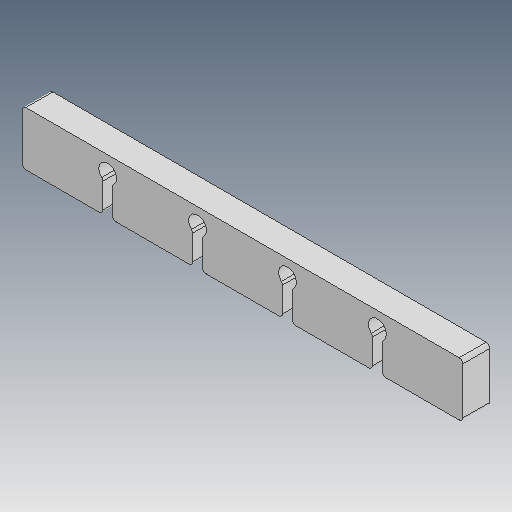
# Autodesk Inventor part: SlipersLåda 211018007
Saved by Autodesk Inventor 2020 (Build 240168000, 168)
## iProperties
Created: 2021-10-19
Part Number: SlipersLåda 211018007
Material: Generic
Document SubType Name: Modeling
Designer: dicpet001
Density: 1 g/cm^3
Appearance: Default
Author: dicpet001
Autodesk Inventor part; units mm, degrees
ref_plane "YZ Plane" through (0, 0, 0) normal (1, 0, 0) x (0, 1, 0)
ref_plane "XZ Plane" through (0, 0, 0) normal (0, 1, 0) x (-1, 0, 0)
ref_plane "XY Plane" through (0, 0, 0) normal (0, 0, 1) x (1, 0, 0)
sketch "Sketch1" plane through (0, 0, 0) normal (0, 0, 1) x (1, 0, 0)
  line L0 (0, 21.5799) -> (0, -21.5799) projected
  line L1 (-172.0799, 0) -> (172.0799, 0) projected
  line L2 (-120.5, 15) -> (120.5, 15)
  line L3 (122.5, 13) -> (122.5, -13)
  line L4 (-122.5, -13) -> (-122.5, 13)
  arc A0 (-21.6071, 2.3273) -> (-28.3929, 2.3273) centre (-25, 6) ccw
  line L5 (-25, 6) -> (-25, -2.9295)
  line L6 (-27.75, 0.8583) -> (-27.75, -13)
  line L7 (-22.25, 0.8583) -> (-22.25, -13)
  arc A1 (-27.75, 0.8583) -> (-28.3929, 2.3273) centre (-29.75, 0.8583) ccw
  arc A2 (-21.6071, 2.3273) -> (-22.25, 0.8583) centre (-20.25, 0.8583) ccw
  arc A3 (-29.75, -15) -> (-27.75, -13) centre (-29.75, -13) ccw
  arc A4 (-22.25, -13) -> (-20.25, -15) centre (-20.25, -13) ccw
  arc A5 (-71.6071, 2.3273) -> (-78.3929, 2.3273) centre (-75, 6) ccw
  line L8 (-75, 6) -> (-75, -2.9295)
  line L9 (-77.75, 0.8583) -> (-77.75, -13)
  line L10 (-72.25, 0.8583) -> (-72.25, -13)
  arc A6 (-77.75, 0.8583) -> (-78.3929, 2.3273) centre (-79.75, 0.8583) ccw
  arc A7 (-71.6071, 2.3273) -> (-72.25, 0.8583) centre (-70.25, 0.8583) ccw
  arc A8 (-79.75, -15) -> (-77.75, -13) centre (-79.75, -13) ccw
  arc A9 (-72.25, -13) -> (-70.25, -15) centre (-70.25, -13) ccw
  line L11 (-29.75, -15) -> (-70.25, -15)
  line L12 (-79.75, -15) -> (-120.5, -15)
  arc A10 (28.3929, 2.3273) -> (21.6071, 2.3273) centre (25, 6) ccw
  line L13 (25, 6) -> (25, -2.9295)
  line L14 (27.75, 0.8583) -> (27.75, -13)
  line L15 (22.25, 0.8583) -> (22.25, -13)
  arc A11 (28.3929, 2.3273) -> (27.75, 0.8583) centre (29.75, 0.8583) ccw
  arc A12 (22.25, 0.8583) -> (21.6071, 2.3273) centre (20.25, 0.8583) ccw
  arc A13 (27.75, -13) -> (29.75, -15) centre (29.75, -13) ccw
  arc A14 (20.25, -15) -> (22.25, -13) centre (20.25, -13) ccw
  line L16 (72.25, 0.8583) -> (72.25, -13)
  arc A15 (72.25, 0.8583) -> (71.6071, 2.3273) centre (70.25, 0.8583) ccw
  arc A16 (70.25, -15) -> (72.25, -13) centre (70.25, -13) ccw
  arc A17 (78.3929, 2.3273) -> (71.6071, 2.3273) centre (75, 6) ccw
  line L17 (77.75, 0.8583) -> (77.75, -13)
  arc A18 (78.3929, 2.3273) -> (77.75, 0.8583) centre (79.75, 0.8583) ccw
  line L18 (75, 6) -> (75, -2.9295)
  arc A19 (77.75, -13) -> (79.75, -15) centre (79.75, -13) ccw
  line L19 (20.25, -15) -> (-20.25, -15)
  line L20 (120.5, -15) -> (79.75, -15)
  line L21 (70.25, -15) -> (29.75, -15)
  arc A20 (-120.5, 15) -> (-122.5, 13) centre (-120.5, 13) ccw
  arc A21 (-122.5, -13) -> (-120.5, -15) centre (-120.5, -13) ccw
  arc A22 (120.5, -15) -> (122.5, -13) centre (120.5, -13) ccw
  arc A23 (122.5, 13) -> (120.5, 15) centre (120.5, 13) ccw
  point P0 (0, 0)
  point P1 (-122.5, 15)
  point P2 (122.5, 15)
  point P3 (-122.5, -15)
  point P4 (-27.75, 1.8242)
  point P5 (-22.25, 1.8242)
  point P6 (-77.75, 1.8242)
  point P7 (-72.25, 1.8242)
  point P8 (27.75, 1.8242)
  point P9 (22.25, 1.8242)
  point P10 (72.25, 1.8242)
  point P11 (77.75, 1.8242)
  dimension "d0" = 245
  dimension "d1" = 30
  dimension "d2" = 10
  dimension "d3" = 25
  dimension "d4" = 6
  dimension "d5" = 5.5
  dimension "d6" = 2
  dimension "d7" = 2
  dimension "d9" = 10
  dimension "d10" = 5.5
  dimension "d11" = 2
  dimension "d12" = 2
  dimension "d13" = 2
  dimension "d14" = 50
  constraints: 56 point on circle, 40 end point, 32 symmetric about line, 25 tangent, 24 centre point, 14 point on line, 12 perpendicular, 7 equal radius, 6 parallel, 1 horizontal, 13 other
  measures "d0" distance of point (-122.5, 15) point (122.5, 15)
  measures "d1" distance of point (-122.5, -15) point (-122.5, 15)
  measures "d2" diameter of A0
  measures "d3" distance from line of L0 L5.start
  measures "d4" distance from line of L1 L5.start
  measures "d5" distance between parallel lines of L7 L6
  measures "d6" radius of A1
  measures "d7" radius of A3
  measures "d9" diameter of A5
  measures "d10" distance between parallel lines of L10 L9
  measures "d11" radius of A6
  measures "d12" radius of A8
  measures "d13" radius of A20
  measures "d14" distance between parallel lines of L5 L8
extrude "Extrusion1" add sketch "Sketch1" against normal blind 15 contours L2 A23 L3 L1 L17 A18 A17 A15 L16 L14 A11 A10 A12 L15 L0 | L0 L1 L7 A2 A0 A1 L6 L10 A7 A5 A6 L9 L4 A20 L2 | L1 L15 A14 L19 L0 | L0 L19 A4 L7 L1 | L1 L9 A8 L12 A21 L4 | L3 A22 L20 A19 L17 L1 | L6 A3 L11 A9 L10 L1 | L1 L16 A16 L21 A13 L14
body "Solid1"
